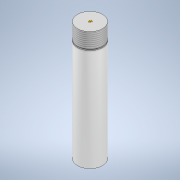
# Autodesk Inventor part: W520superior
Saved by Autodesk Inventor 2020 (Build 240168000, 168)
## iProperties
Created: 2021-10-16
Part Number: W520superior
Material: Genérico
Document SubType Name: Modeling
Designer: DANIEL
Density: 1 g/cm^3
Appearance: Valor por defecto
Author: DANIEL
Autodesk Inventor part; units mm, degrees
ref_plane "YZ Plane" through (0, 0, 0) normal (1, 0, 0) x (0, 1, 0)
ref_plane "XZ Plane" through (0, 0, 0) normal (0, 1, 0) x (-1, 0, 0)
sketch "Boceto1" plane through (0, 0, 0) normal (0, 1, 0) x (-1, 0, 0)
  circle A0 centre (0, 0) radius 11
  dimension "d0" = 22
  constraints: 1 centre point, 1 coincident
  measures "d0" diameter of A0
extrude "Extrusión1" add sketch "Boceto1" along normal blind 105
ref_plane "Plano de trabajo1" through (0, 91.5, 0) normal (0, 1, 0) x (1, 0, 0)
sketch "Boceto2" plane through (0, 91.5, 0) normal (0, 1, 0) x (1, 0, 0)
  circle A0 centre (0, 0) radius 11
  circle A1 centre (0, 0) radius 10
  dimension "d4" = 20
  constraints: 2 centre point, 2 coincident
  measures "d4" diameter of A1
extrude "Extrusión2" cut sketch "Boceto2" against normal blind 1
thread "Rosca1" size "M22x1.5" class "6g" standard "ANSI Metric M Profile" full length
